Autodesk Inventor part; units mm, degrees
(part 3 of 4)
  line L1036 (-8.35, 24.45) -> (-11.15, 24.45)
  line L1037 (-11.15, 43.95) -> (-8.35, 43.95)
  line L1038 (-9.5, 42.651) -> (-9.5, 43.15)
  line L1039 (-10, 43.15) -> (-10, 42.517)
  line L1040 (-10, 43.15) -> (-9.5, 42.45) construction
  line L1041 (-10, 42.45) -> (-9.5, 43.15) construction
  arc A311 (-9.5, 42.651) -> (-9.433, 42.401) centre (-9, 42.651) ccw
  arc A312 (-10, 42.517) -> (-9.933, 42.267) centre (-9.5, 42.517) ccw
  line L1042 (-8.35, 43.95) -> (-8.35, 43.15)
  line L1043 (-8.35, 43.15) -> (-9.5, 43.15)
  line L1044 (-9.5, 43.15) -> (-10, 43.15)
  line L1045 (-9.75, 48.75) -> (-9.75, 43.95)
  line L1046 (-10, 43.15) -> (-11.15, 43.15)
  line L1047 (-11.15, 43.15) -> (-11.15, 43.95)
  line L1048 (-9.933, 22.767) -> (-2.2258, 9.4177)
  line L1049 (-1.7258, 9.5516) -> (-9.433, 22.901)
  line L1050 (-9.5335, 23.075) -> (-9.9665, 22.825)
  line L1051 (-9.9665, 22.825) -> (-1.6923, 9.4936) construction
  line L1052 (-2.1253, 9.2436) -> (-9.5335, 23.075) construction
  line L1053 (-9.5, 23.65) -> (-10, 23.65)
  line L1054 (-9.5, 23.151) -> (-9.5, 23.65)
  line L1055 (-10, 23.65) -> (-10, 23.017)
  line L1056 (-10, 23.65) -> (-9.5, 22.95) construction
  line L1057 (-10, 22.95) -> (-9.5, 23.65) construction
  line L1058 (-10, 22.95) -> (-9.5, 22.95)
  arc A313 (-9.5, 23.151) -> (-9.433, 22.901) centre (-9, 23.151) ccw
  arc A314 (-10, 23.017) -> (-9.933, 22.767) centre (-9.5, 23.017) ccw
  line L1059 (-0.2828, -49.3267) -> (2.4885, -54.1267)
  line L1060 (-0.2081, -55.5191) -> (0.2919, -52.6564) construction
  line L1061 (-0.2081, -52.6564) -> (0.2919, -55.5191) construction
  line L1062 (0.2919, -52.7233) -> (0.2919, -55.5191)
  circle A315 centre (0.0419, -55.5191) radius 0.75
  line L1063 (-0.2081, -55.5191) -> (-0.2081, -52.8573)
  arc A316 (-1.9445, -52.117) -> (-2.0115, -51.867) centre (-2.4445, -52.117) ccw
  arc A317 (-1.4445, -51.983) -> (-1.5115, -51.733) centre (-1.9445, -51.983) ccw
  arc A318 (-0.2081, -52.8573) -> (-0.2751, -52.6073) centre (-0.7081, -52.8573) ccw
  arc A319 (0.2919, -52.7233) -> (0.2249, -52.4733) centre (-0.2081, -52.7233) ccw
  line L1064 (2.089, -54.4347) -> (-0.3833, -49.1526) construction
  arc A320 (-0.3498, -49.0767) -> (-0.2828, -49.3267) centre (0.1502, -49.0767) ccw
  arc A321 (-0.8498, -49.2107) -> (-0.7828, -49.4607) centre (-0.3498, -49.2107) ccw
  arc A322 (-2.1588, -49.2107) -> (-2.0918, -49.4607) centre (-1.6588, -49.2107) ccw
  arc A323 (-1.6588, -49.0767) -> (-1.5918, -49.3267) centre (-1.1588, -49.0767) ccw
  line L1065 (-0.1746, -52.7814) -> (-1.6923, -49.1526) construction
  line L1066 (2.5555, -60.0187) -> (2.0555, -60.0187)
  circle A324 centre (2.3055, -60.0191) radius 0.75
  line L1067 (0.2919, -55.5191) -> (-0.2081, -55.5191)
  line L1068 (-4.2704, -49.3778) -> (-3.7751, -50.2357)
  line L1069 (-4.1686, -50.5541) -> (-4.3798, -49.1883) construction
  arc A325 (-4.3374, -49.1278) -> (-4.2704, -49.3778) centre (-3.8374, -49.1278) ccw
  arc A326 (-3.7081, -50.4857) -> (-3.7751, -50.2357) centre (-4.2081, -50.4857) ccw
  arc A327 (-3.4678, -49.2107) -> (-3.4008, -49.4607) centre (-2.9678, -49.2107) ccw
  arc A328 (-2.9678, -49.0767) -> (-2.9008, -49.3267) centre (-2.4678, -49.0767) ccw
  arc A329 (-4.2081, -50.6197) -> (-4.2751, -50.3697) centre (-4.7081, -50.6197) ccw
  arc A330 (2.5555, -54.3767) -> (2.4885, -54.1267) centre (2.0555, -54.3767) ccw
  arc A331 (2.0555, -54.5107) -> (1.9885, -54.2607) centre (1.5555, -54.5107) ccw
  line L1070 (-3.7081, -55.5191) -> (-4.2081, -55.5191)
  circle A332 centre (-3.9581, -55.5191) radius 0.75
  line L1071 (-1.9445, -60.0191) -> (-1.4445, -60.0191)
  circle A333 centre (-1.6945, -60.0191) radius 0.75
  line L1072 (-5.9445, -60.0191) -> (-5.4445, -60.0191)
  circle A334 centre (-5.6945, -60.0191) radius 0.75
  line L1073 (-8.35, -53.55) -> (-11.15, -53.55)
  line L1074 (-9.4445, -54.35) -> (-8.35, -54.35)
  line L1075 (-8.35, -54.35) -> (-8.35, -53.55)
  line L1076 (-11.15, -54.35) -> (-9.9295, -54.35)
  line L1077 (-11.15, -53.55) -> (-11.15, -54.35)
  line L1078 (-19.7751, -52.6073) -> (-21.5918, -49.4607)
  line L1079 (-23.2081, -50.4857) -> (-23.2081, -55.5191)
  line L1080 (-23.7081, -55.5191) -> (-23.7081, -50.6197)
  line L1081 (-23.7081, -55.5191) -> (-23.2081, -50.4326) construction
  line L1082 (-23.7081, -50.4326) -> (-23.2081, -55.5191) construction
  line L1083 (-22.9008, -49.4607) -> (-21.5115, -51.867)
  line L1084 (-20.9445, -60.0191) -> (-20.9445, -51.983)
  line L1085 (-21.4445, -51.916) -> (-20.9445, -60.0191) construction
  line L1086 (-21.4445, -60.0191) -> (-20.9445, -51.916) construction
  line L1087 (-21.4445, -52.117) -> (-21.4445, -60.0191)
  line L1088 (-24.3128, -49.4383) -> (-23.2356, -50.3041) construction
  line L1089 (-23.7751, -50.3697) -> (-24.2704, -49.5118)
  line L1090 (-25.5188, -49.4607) -> (-25.5115, -49.4733)
  line L1091 (-24.9445, -60.0191) -> (-24.9445, -49.5893)
  line L1092 (-25.4445, -49.7233) -> (-25.4445, -60.0191)
  line L1093 (-24.9445, -49.5223) -> (-25.4445, -60.0191) construction
  line L1094 (-24.9445, -60.0191) -> (-25.4445, -49.5223) construction
  line L1095 (-17.4445, -60.0187) -> (-17.4445, -54.5107)
  line L1096 (-16.9445, -54.3767) -> (-16.9445, -60.0187)
  line L1097 (-17.4445, -54.3101) -> (-16.9445, -60.0187) construction
  line L1098 (-17.4445, -60.0187) -> (-16.9445, -54.3101) construction
  line L1099 (-29.4295, -60.0191) -> (-29.4295, -54.35)
  line L1100 (-28.9445, -60.0191) -> (-29.4295, -60.0191)
  circle A335 centre (-29.1945, -60.0191) radius 0.75
  line L1101 (-29.4295, -60.0191) -> (-28.9832, -54.35) construction
  line L1102 (-29.4295, -54.35) -> (-28.9445, -54.35)
  line L1103 (-28.9445, -54.35) -> (-28.9445, -60.0191)
  line L1104 (-29.4295, -54.2285) -> (-28.9445, -60.0191) construction
  arc A336 (-24.9445, -49.5893) -> (-25.0115, -49.3393) centre (-25.4445, -49.5893) ccw
  arc A337 (-24.3374, -49.2618) -> (-24.2704, -49.5118) centre (-23.8374, -49.2618) ccw
  arc A338 (-25.0858, -49.0767) -> (-25.0188, -49.3267) centre (-24.5858, -49.0767) ccw
  arc A339 (-25.4445, -49.7233) -> (-25.5115, -49.4733) centre (-25.9445, -49.7233) ccw
  arc A340 (-25.5858, -49.2107) -> (-25.5188, -49.4607) centre (-25.0858, -49.2107) ccw
  line L1105 (-22.9343, -49.4026) -> (-20.978, -51.791) construction
  line L1106 (-21.0115, -51.733) -> (-22.4008, -49.3267)
  line L1107 (-21.411, -52.041) -> (-22.5013, -49.1526) construction
  line L1108 (-17.5115, -54.2607) -> (-20.2828, -49.4607)
  line L1109 (-22.9678, -49.2107) -> (-22.9678, -8.0651)
  line L1110 (-22.9678, -49.2776) -> (-22.4678, -7.8641) construction
  line L1111 (-22.9678, -7.8641) -> (-22.4678, -49.2776) construction
  line L1112 (-22.4678, -7.9311) -> (-22.4678, -49.0767)
  line L1113 (-21.6588, 9.1677) -> (-21.6588, -49.2107)
  line L1114 (-21.1588, -49.0767) -> (-21.1588, 9.3016)
  line L1115 (-21.6588, -49.2776) -> (-21.1588, 9.3686) construction
  line L1116 (-20.3498, -49.2107) -> (-20.3498, 26.4004)
  line L1117 (-19.8498, 26.5344) -> (-19.8498, -49.0767)
  line L1118 (-21.6588, 9.3686) -> (-21.1588, -49.2776) construction
  line L1119 (-21.6253, -49.4026) -> (-19.2416, -52.5314) construction
  line L1120 (-20.3163, -49.4026) -> (-16.978, -54.1847) construction
  line L1121 (-21.0918, -49.3267) -> (-19.2751, -52.4733)
  line L1122 (-25.5858, -42.4055) -> (-25.5858, -49.2107)
  line L1123 (-25.0858, -49.0767) -> (-25.0858, -42.2693)
  line L1124 (-25.5858, -49.2776) -> (-25.0858, -42.2012) construction
  line L1125 (-25.5858, -42.2012) -> (-25.0858, -49.2776) construction
  line L1126 (-29.4309, -35.7355) -> (-25.6549, -42.1519)
  line L1127 (-25.5513, -42.328) -> (-29.0345, -35.4232) construction
  line L1128 (-25.1549, -42.0157) -> (-28.9309, -35.5993)
  arc A341 (-25.5858, -42.4055) -> (-25.6549, -42.1519) centre (-26.0858, -42.4055) ccw
  arc A342 (-25.0858, -42.2693) -> (-25.1549, -42.0157) centre (-25.5858, -42.2693) ccw
  line L1129 (-29.4655, -35.6768) -> (-25.1203, -42.0744) construction
  arc A343 (-29.5, -35.4819) -> (-29.4309, -35.7355) centre (-29, -35.4819) ccw
  arc A344 (-29, -35.3457) -> (-28.9309, -35.5993) centre (-28.5, -35.3457) ccw
  line L1130 (-29, -35.3457) -> (-29, -34.85)
  line L1131 (-29.5, -35.55) -> (-29, -34.85) construction
  line L1132 (-29.5, -34.85) -> (-29, -35.55) construction
  line L1133 (-29, -34.85) -> (-29.5, -34.85)
  line L1134 (-29.5, -34.85) -> (-29.5, -35.4819)
  line L1135 (-25.0115, -49.3393) -> (-25.0188, -49.3267)
  line L1136 (-24.3374, -25.1978) -> (-24.3374, -49.2618)
  line L1137 (-23.8374, -49.1278) -> (-23.8374, -25.0639)
  line L1138 (-24.3374, -25.002) -> (-23.8374, -49.3098) construction
  line L1139 (-24.3374, -49.3098) -> (-23.8374, -25.002) construction
  arc A345 (-23.8374, -25.0639) -> (-23.9043, -24.814) centre (-24.3374, -25.0639) ccw
  arc A346 (-24.3374, -25.1978) -> (-24.4043, -24.9479) centre (-24.8374, -25.1978) ccw
  line L1140 (-30.65, -34.85) -> (-29.5, -34.85)
  line L1141 (-29, -34.85) -> (-27.85, -34.85)
  line L1142 (-30.65, -34.05) -> (-30.65, -34.85)
  line L1143 (-27.85, -34.05) -> (-30.65, -34.05)
  line L1144 (-27.85, -34.85) -> (-27.85, -34.05)
  arc A347 (-29.5, -15.983) -> (-29.4331, -16.2329) centre (-29, -15.983) ccw
  line L1145 (-29.0335, -15.9251) -> (-29.4665, -16.1749)
  line L1146 (-29.4331, -16.2329) -> (-24.4043, -24.9479)
  line L1147 (-29.4665, -16.1749) -> (-23.8679, -24.8771) construction
  line L1148 (-24.301, -25.127) -> (-29.0335, -15.9251) construction
  line L1149 (-23.9043, -24.814) -> (-28.9331, -16.099)
  line L1150 (-29.5, -16.05) -> (-29, -16.05)
  arc A348 (-29, -15.8491) -> (-28.9331, -16.099) centre (-28.5, -15.8491) ccw
  line L1151 (-29.25, -15.35) -> (-29.25, -16.05)
  line L1152 (-29.5, -15.35) -> (-29, -16.05) construction
  line L1153 (-29.5, -16.05) -> (-29, -15.35) construction
  line L1154 (-29, -15.35) -> (-29.5, -15.35)
  line L1155 (-30.65, -15.35) -> (-29.5, -15.35)
  line L1156 (-27.85, -14.55) -> (-30.65, -14.55)
  line L1157 (-30.65, -14.55) -> (-30.65, -15.35)
  line L1158 (-29.5, -15.35) -> (-29.5, -15.983)
  arc A349 (-22.4678, -7.9311) -> (-22.5348, -7.6811) centre (-22.9678, -7.9311) ccw
  arc A350 (-22.9678, -8.0651) -> (-23.0348, -7.8151) centre (-23.4678, -8.0651) ccw
  line L1159 (-29, -15.8491) -> (-29, -15.35)
  line L1160 (-29, -15.35) -> (-27.85, -15.35)
  line L1161 (-27.85, -15.35) -> (-27.85, -14.55)
  line L1162 (-29.433, 3.267) -> (-23.0348, -7.8151)
  line L1163 (-22.5348, -7.6811) -> (-28.933, 3.401)
  line L1164 (-29.0335, 3.575) -> (-29.4665, 3.325)
  line L1165 (-29.4665, 3.325) -> (-22.5013, -7.7391) construction
  line L1166 (-22.9343, -7.9891) -> (-29.0335, 3.575) construction
  line L1167 (-29.5, 3.45) -> (-29, 3.45)
  arc A351 (-29.5, 3.517) -> (-29.433, 3.267) centre (-29, 3.517) ccw
  line L1168 (-27.85, 4.15) -> (-27.85, 4.95)
  line L1169 (-29, 4.15) -> (-27.85, 4.15)
  line L1170 (-29, 3.651) -> (-29, 4.15)
  line L1171 (-29, 4.15) -> (-29.5, 4.15)
  arc A352 (-29, 3.651) -> (-28.933, 3.401) centre (-28.5, 3.651) ccw
  line L1172 (-29.5, 4.15) -> (-29.5, 3.517)
  line L1173 (-27.85, 4.95) -> (-30.65, 4.95)
  line L1174 (-30.65, 4.95) -> (-30.65, 4.15)
  line L1175 (-30.65, 4.15) -> (-29.5, 4.15)
  line L1176 (-21.6253, 9.2436) -> (-21.1923, 9.4936)
  arc A353 (-21.6588, 9.1677) -> (-21.7258, 9.4177) centre (-22.1588, 9.1677) ccw
  arc A354 (-21.1588, 9.3016) -> (-21.2258, 9.5516) centre (-21.6588, 9.3016) ccw
  line L1177 (-29.433, 42.267) -> (-20.4168, 26.6504)
  line L1178 (-20.3163, 26.4764) -> (-19.8833, 26.7264)
  line L1179 (-19.9168, 26.7844) -> (-28.933, 42.401)
  line L1180 (-29.4665, 42.325) -> (-19.8833, 26.7264) construction
  line L1181 (-20.3163, 26.4764) -> (-29.0335, 42.575) construction
  arc A355 (-19.8498, 26.5344) -> (-19.9168, 26.7844) centre (-20.3498, 26.5344) ccw
  arc A356 (-20.3498, 26.4004) -> (-20.4168, 26.6504) centre (-20.8498, 26.4004) ccw
  line L1182 (-29, 23.65) -> (-27.85, 23.65)
  line L1183 (-27.85, 23.65) -> (-27.85, 24.45)
  line L1184 (-30.65, 24.45) -> (-30.65, 23.65)
  line L1185 (-30.65, 23.65) -> (-29.5, 23.65)
  line L1186 (-27.85, 24.45) -> (-30.65, 24.45)
  line L1187 (-30.65, 43.95) -> (-27.85, 43.95)
  line L1188 (-29, 42.651) -> (-29, 43.15)
  line L1189 (-29.5, 43.15) -> (-29.5, 42.517)
  line L1190 (-29.5, 43.15) -> (-29, 42.45) construction
  line L1191 (-29.5, 42.45) -> (-29, 43.15) construction
  arc A357 (-29, 42.651) -> (-28.933, 42.401) centre (-28.5, 42.651) ccw
  arc A358 (-29.5, 42.517) -> (-29.433, 42.267) centre (-29, 42.517) ccw
  line L1192 (-27.85, 43.95) -> (-27.85, 43.15)
  line L1193 (-27.85, 43.15) -> (-29, 43.15)
  line L1194 (-29, 43.15) -> (-29.5, 43.15)
  line L1195 (-29.25, 48.75) -> (-29.25, 43.95)
  line L1196 (-29.5, 43.15) -> (-30.65, 43.15)
  line L1197 (-30.65, 43.15) -> (-30.65, 43.95)
  line L1198 (-29.433, 22.767) -> (-21.7258, 9.4177)
  line L1199 (-21.2258, 9.5516) -> (-28.933, 22.901)
  line L1200 (-29.0335, 23.075) -> (-29.4665, 22.825)
  line L1201 (-29.4665, 22.825) -> (-21.1923, 9.4936) construction
  line L1202 (-21.6253, 9.2436) -> (-29.0335, 23.075) construction
  line L1203 (-29, 23.65) -> (-29.5, 23.65)
  line L1204 (-29, 23.151) -> (-29, 23.65)
  line L1205 (-29.5, 23.65) -> (-29.5, 23.017)
  line L1206 (-29.5, 23.65) -> (-29, 22.95) construction
  line L1207 (-29.5, 22.95) -> (-29, 23.65) construction
  line L1208 (-29.5, 22.95) -> (-29, 22.95)
  arc A359 (-29, 23.151) -> (-28.933, 22.901) centre (-28.5, 23.151) ccw
  arc A360 (-29.5, 23.017) -> (-29.433, 22.767) centre (-29, 23.017) ccw
  line L1209 (-19.7828, -49.3267) -> (-17.0115, -54.1267)
  line L1210 (-19.7081, -55.5191) -> (-19.2081, -52.6564) construction
  line L1211 (-19.7081, -52.6564) -> (-19.2081, -55.5191) construction
  line L1212 (-19.2081, -52.7233) -> (-19.2081, -55.5191)
  circle A361 centre (-19.4581, -55.5191) radius 0.75
  line L1213 (-19.7081, -55.5191) -> (-19.7081, -52.8573)
  arc A362 (-21.4445, -52.117) -> (-21.5115, -51.867) centre (-21.9445, -52.117) ccw
  arc A363 (-20.9445, -51.983) -> (-21.0115, -51.733) centre (-21.4445, -51.983) ccw
  arc A364 (-19.7081, -52.8573) -> (-19.7751, -52.6073) centre (-20.2081, -52.8573) ccw
  arc A365 (-19.2081, -52.7233) -> (-19.2751, -52.4733) centre (-19.7081, -52.7233) ccw
  line L1214 (-17.411, -54.4347) -> (-19.8833, -49.1526) construction
  arc A366 (-19.8498, -49.0767) -> (-19.7828, -49.3267) centre (-19.3498, -49.0767) ccw
  arc A367 (-20.3498, -49.2107) -> (-20.2828, -49.4607) centre (-19.8498, -49.2107) ccw
  arc A368 (-21.6588, -49.2107) -> (-21.5918, -49.4607) centre (-21.1588, -49.2107) ccw
  arc A369 (-21.1588, -49.0767) -> (-21.0918, -49.3267) centre (-20.6588, -49.0767) ccw
  line L1215 (-19.6746, -52.7814) -> (-21.1923, -49.1526) construction
  line L1216 (-16.9445, -60.0187) -> (-17.4445, -60.0187)
  circle A370 centre (-17.1945, -60.0191) radius 0.75
  line L1217 (-19.2081, -55.5191) -> (-19.7081, -55.5191)
  line L1218 (-23.7704, -49.3778) -> (-23.2751, -50.2357)
  line L1219 (-23.6686, -50.5541) -> (-23.8798, -49.1883) construction
  arc A371 (-23.8374, -49.1278) -> (-23.7704, -49.3778) centre (-23.3374, -49.1278) ccw
  arc A372 (-23.2081, -50.4857) -> (-23.2751, -50.2357) centre (-23.7081, -50.4857) ccw
  arc A373 (-22.9678, -49.2107) -> (-22.9008, -49.4607) centre (-22.4678, -49.2107) ccw
  arc A374 (-22.4678, -49.0767) -> (-22.4008, -49.3267) centre (-21.9678, -49.0767) ccw
  arc A375 (-23.7081, -50.6197) -> (-23.7751, -50.3697) centre (-24.2081, -50.6197) ccw
  arc A376 (-16.9445, -54.3767) -> (-17.0115, -54.1267) centre (-17.4445, -54.3767) ccw
  arc A377 (-17.4445, -54.5107) -> (-17.5115, -54.2607) centre (-17.9445, -54.5107) ccw
  line L1220 (-23.2081, -55.5191) -> (-23.7081, -55.5191)
  circle A378 centre (-23.4581, -55.5191) radius 0.75
  line L1221 (-21.4445, -60.0191) -> (-20.9445, -60.0191)
  circle A379 centre (-21.1945, -60.0191) radius 0.75
  line L1222 (-25.4445, -60.0191) -> (-24.9445, -60.0191)
  circle A380 centre (-25.1945, -60.0191) radius 0.75
  line L1223 (-27.85, -53.55) -> (-30.65, -53.55)
  line L1224 (-28.9445, -54.35) -> (-27.85, -54.35)
  line L1225 (-27.85, -54.35) -> (-27.85, -53.55)
  line L1226 (-30.65, -54.35) -> (-29.4295, -54.35)
  line L1227 (-30.65, -53.55) -> (-30.65, -54.35)
  point P0 (27.85, 43.15)
  point P1 (38.4002, -11.3381)
  point P2 (39.8528, -51.7937)
  point P3 (41.3055, -57.1644)
  point P4 (39.0419, -54.0877)
  point P5 (38.0666, -50.967)
  point P6 (36.5438, -50.5968)
  point P7 (37.3055, -55.9676)
  point P8 (37.0912, -19.9545)
  point P9 (35.7822, -28.5709)
  point P10 (35.0419, -52.9758)
  point P11 (34.7258, -49.8712)
  point P12 (33.3055, -54.7707)
  point P13 (33.1642, -45.7394)
  point P14 (34.4126, -37.1559)
  point P15 (33.8251, 34.5257)
  point P16 (29.25, 42.8)
  point P17 (33.1706, 16.1593)
  point P18 (31.8328, -20.526)
  point P19 (31.2071, -38.8756)
  point P20 (32.5161, -2.2071)
  point P21 (29.25, 23.3)
  point P22 (29.25, -15.7)
  point P23 (29.25, -35.2)
  point P24 (29.3055, -57.0343)
  point P25 (29.1945, 57.0343)
  point P26 (21.1945, 55.9676)
  point P27 (17.1945, 57.1644)
  point P28 (25.1945, 54.7707)
  point P29 (23.4581, 52.9758)
  point P30 (23.7742, 49.8712)
  point P31 (18.6472, 51.7937)
  point P32 (19.4581, 54.0877)
  point P33 (21.9562, 50.5968)
  point P34 (20.4334, 50.967)
  point P35 (25.3358, 45.7394)
  point P36 (24.0874, 37.1559)
  point P37 (27.2929, 38.8756)
  point P38 (29.25, 35.2)
  point P39 (29.25, 15.7)
  point P40 (25.9839, 2.2071)
  point P41 (20.0998, 11.3381)
  point P42 (21.4088, 19.9545)
  point P43 (22.7178, 28.5709)
  point P44 (25.3294, -16.1593)
  point P45 (29.25, -23.3)
  point P46 (24.6749, -34.5257)
  point P47 (29.25, -42.8)
  point P48 (26.6672, 20.526)
  point P49 (9.6945, 57.0343)
  point P50 (1.6945, 55.9676)
  point P51 (-2.3055, 57.1644)
  point P52 (5.6945, 54.7707)
  point P53 (3.9581, 52.9758)
  point P54 (4.2742, 49.8712)
  point P55 (-0.8528, 51.7937)
  point P56 (-0.0419, 54.0877)
  point P57 (2.4562, 50.5968)
  point P58 (0.9334, 50.967)
  point P59 (5.8358, 45.7394)
  point P60 (4.5874, 37.1559)
  point P61 (7.7929, 38.8756)
  point P62 (9.75, 35.2)
  point P63 (9.75, 15.7)
  point P64 (6.4839, 2.2071)
  point P65 (0.5998, 11.3381)
  point P66 (1.9088, 19.9545)
  point P67 (3.2178, 28.5709)
  point P68 (5.8294, -16.1593)
  point P69 (9.75, -23.3)
  point P70 (5.1749, -34.5257)
  point P71 (9.75, -42.8)
  point P72 (7.1672, 20.526)
  point P73 (-9.8055, 57.0343)
  point P74 (-17.8055, 55.9676)
  point P75 (-21.8055, 57.1644)
  point P76 (-13.8055, 54.7707)
  point P77 (-15.5419, 52.9758)
  point P78 (-15.2258, 49.8712)
  point P79 (-20.3528, 51.7937)
  point P80 (-19.5419, 54.0877)
  point P81 (-17.0438, 50.5968)
  point P82 (-18.5666, 50.967)
  point P83 (-13.6642, 45.7394)
  point P84 (-14.9126, 37.1559)
  point P85 (-11.7071, 38.8756)
  point P86 (-9.75, 35.2)
  point P87 (-9.75, 15.7)
  point P88 (-13.0161, 2.2071)
  point P89 (-18.9002, 11.3381)
  point P90 (-17.5912, 19.9545)
  point P91 (-16.2822, 28.5709)
  point P92 (-13.6706, -16.1593)
  point P93 (-9.75, -23.3)
  point P94 (-14.3251, -34.5257)
  point P95 (-9.75, -42.8)
  point P96 (-12.3328, 20.526)
  point P97 (-29.3055, 57.0343)
  point P98 (-37.3055, 55.9676)
  point P99 (-41.3055, 57.1644)
  point P100 (-33.3055, 54.7707)
  point P101 (-35.0419, 52.9758)
  point P102 (-34.7258, 49.8712)
  point P103 (-39.8528, 51.7937)
  point P104 (-39.0419, 54.0877)
  point P105 (-36.5438, 50.5968)
  point P106 (-38.0666, 50.967)
  point P107 (-33.1642, 45.7394)
  point P108 (-34.4126, 37.1559)
  point P109 (-31.2071, 38.8756)
  point P110 (-29.25, 35.2)
  point P111 (-29.25, 15.7)
  point P112 (-32.5161, 2.2071)
  point P113 (-38.4002, 11.3381)
  point P114 (-37.0912, 19.9545)
  point P115 (-35.7822, 28.5709)
  point P116 (-33.1706, -16.1593)
  point P117 (-29.25, -23.3)
  point P118 (-33.8251, -34.5257)
  point P119 (-29.25, -42.8)
  point P120 (-31.8328, 20.526)
  point P121 (17.8055, -55.9676)
  point P122 (15.5419, -52.9758)
  point P123 (18.5666, -50.967)
  point P124 (17.0438, -50.5968)
  point P125 (13.8055, -54.7707)
  point P126 (9.8055, -57.0343)
  point P127 (17.5912, -19.9545)
  point P128 (18.9002, -11.3381)
  point P129 (13.6642, -45.7394)
  point P130 (11.7071, -38.8756)
  point P131 (9.75, -35.2)
  point P132 (16.2822, -28.5709)
  point P133 (14.9126, -37.1559)
  point P134 (12.3328, -20.526)
  point P135 (9.75, -15.7)
  point P136 (13.0161, -2.2071)
  point P137 (14.3251, 34.5257)
  point P138 (9.75, 42.8)
  point P139 (13.6706, 16.1593)
  point P140 (9.75, 23.3)
  point P141 (19.5419, -54.0877)
  point P142 (20.3528, -51.7937)
  point P143 (21.8055, -57.1644)
  point P144 (15.2258, -49.8712)
  point P145 (-1.6945, -55.9676)
  point P146 (-3.9581, -52.9758)
  point P147 (-0.9334, -50.967)
  point P148 (-2.4562, -50.5968)
  point P149 (-5.6945, -54.7707)
  point P150 (-9.6945, -57.0343)
  point P151 (-1.9088, -19.9545)
  point P152 (-0.5998, -11.3381)
  point P153 (-5.8358, -45.7394)
  point P154 (-7.7929, -38.8756)
  point P155 (-9.75, -35.2)
  point P156 (-3.2178, -28.5709)
  point P157 (-4.5874, -37.1559)
  point P158 (-7.1672, -20.526)
  point P159 (-9.75, -15.7)
  point P160 (-6.4839, -2.2071)
  point P161 (-5.1749, 34.5257)
  point P162 (-9.75, 42.8)
  point P163 (-5.8294, 16.1593)
  point P164 (-9.75, 23.3)
  point P165 (0.0419, -54.0877)
  point P166 (0.8528, -51.7937)
  point P167 (2.3055, -57.1644)
  point P168 (-4.2742, -49.8712)
  point P169 (-21.1945, -55.9676)
  point P170 (-23.4581, -52.9758)
  point P171 (-20.4334, -50.967)
  point P172 (-21.9562, -50.5968)
  point P173 (-25.1945, -54.7707)
  point P174 (-29.1945, -57.0343)
  point P175 (-21.4088, -19.9545)
  point P176 (-20.0998, -11.3381)
  point P177 (-25.3358, -45.7394)
  point P178 (-27.2929, -38.8756)
  point P179 (-29.25, -35.2)
  point P180 (-22.7178, -28.5709)
  point P181 (-24.0874, -37.1559)
  point P182 (-26.6672, -20.526)
  point P183 (-29.25, -15.7)
  point P184 (-25.9839, -2.2071)
  point P185 (-24.6749, 34.5257)
  point P186 (-29.25, 42.8)
  point P187 (-25.3294, 16.1593)
  point P188 (-29.25, 23.3)
  point P189 (-19.4581, -54.0877)
  point P190 (-18.6472, -51.7937)
  point P191 (-17.1945, -57.1644)
  point P192 (-23.7742, -49.8712)
  dimension "d149" = 0.5
  dimension "d150" = 0.5
  dimension "d151" = 0.5
  dimension "d152" = 0.5
  dimension "d153" = 0.5
  dimension "d154" = 0.5
  dimension "d155" = 0.5
  dimension "d157" = 0.5
  dimension "d161" = 1.5
  dimension "d162" = 1.5
  dimension "d163" = 1.5
  dimension "d164" = 1.5
  dimension "d165" = 1.5
  dimension "d166" = 1.5
  dimension "d180" = 0.5
  dimension "d184" = 0.5
  dimension "d185" = 0.5
  dimension "d186" = 0.5
  dimension "d188" = 0.5
  dimension "d189" = 0.5
  dimension "d190" = 0.5
  dimension "d191" = 0.5
  dimension "d192" = 0.5
  dimension "d193" = 0.5
  dimension "d194" = 0.5
  dimension "d195" = 0.5
  dimension "d196" = 0.5
  dimension "d197" = 0.5
  dimension "d198" = 0.5
  dimension "d199" = 0.5
  dimension "d201" = 0.5
  dimension "d433" = 0.5
  dimension "d434" = 0.5
  dimension "d435" = 0.5
  dimension "d436" = 0.5
  dimension "d437" = 0.5
  dimension "d438" = 0.5
  dimension "d439" = 0.5
  dimension "d440" = 0.5
  dimension "d441" = 1.5
  dimension "d442" = 1.5
  dimension "d443" = 1.5
  dimension "d444" = 1.5
  dimension "d445" = 1.5
  dimension "d446" = 1.5
  dimension "d447" = 0.5
  dimension "d448" = 0.5
  dimension "d449" = 0.5
  dimension "d450" = 0.5
  dimension "d451" = 0.5
  dimension "d452" = 0.5
  dimension "d453" = 0.5
  dimension "d454" = 0.5
  dimension "d455" = 0.5
  dimension "d456" = 0.5
  dimension "d457" = 0.5
  dimension "d458" = 0.5
  dimension "d459" = 0.5
  dimension "d460" = 0.5
  dimension "d461" = 0.5
  dimension "d462" = 0.5
  dimension "d463" = 0.5
  dimension "d464" = 0.5
  dimension "d465" = 0.5
  constraints: 2400 end point, 640 point on circle, 592 point on line, 368 centre point, 364 midpoint, 320 tangent, 190 parallel, 120 equal radius, 57 perpendicular, 20 horizontal, 6 coincident, 4 collinear, 4 vertical
  measures "d149" distance of L8.start L7.end
  measures "d150" distance of L13.start L12.end
  measures "d151" distance of L18.start L17.end
  measures "d152" distance of L22.start L21.end
  measures "d153" distance of L25.end L26.start
  measures "d154" distance of L28.end L27.end
  measures "d155" distance of L34.end L35.start
  measures "d157" distance of L44.start L43.end
  measures "d161" diameter of A6
  measures "d162" diameter of A7
  measures "d163" diameter of A8
  measures "d164" diameter of A9
  measures "d165" diameter of A10
  measures "d166" diameter of A11
  measures "d180" radius of A31
  measures "d184" distance of L66.end L66.start
  measures "d185" radius of A32
  measures "d186" distance of L78.end L79.start
  measures "d188" distance of L82.end L82.start
  measures "d189" radius of A36
  measures "d190" distance of L93.end L94.start
  measures "d191" distance of L97.end L98.start
  measures "d192" distance of L102.end L103.start
  measures "d193" radius of A38
  measures "d194" radius of A40
  measures "d195" radius of A42
  measures "d196" distance of L118.end L118.start
  measures "d197" distance of L123.end L123.start
  measures "d198" distance of L126.end L126.start
  measures "d199" distance of L132.end L133.start
  measures "d201" distance of L156.start L159.start
  measures "d433" distance of L820.start L914.end
  measures "d434" distance of L797.start L798.end
  measures "d435" distance of L911.start L910.end
  measures "d436" distance of L819.start L915.end
  measures "d437" distance of L805.end L807.start
  measures "d438" distance of L785.end L786.start
  measures "d439" distance of L818.end L815.start
  measures "d440" distance of L782.start L781.end
  measures "d441" diameter of A278
  measures "d442" diameter of A287
  measures "d443" diameter of A269
  measures "d444" diameter of A286
  measures "d445" diameter of A288
  measures "d446" diameter of A243
  measures "d447" radius of A284
  measures "d448" distance of L878.end L878.start
  measures "d449" radius of A263
  measures "d450" distance of L890.end L891.start
  measures "d451" distance of L901.end L902.start
  measures "d452" radius of A262
  measures "d453" distance of L847.end L848.start
  measures "d454" distance of L829.end L827.start
  measures "d455" distance of L865.end L866.start
  measures "d456" radius of A257
  measures "d457" radius of A253
  measures "d458" radius of A250
  measures "d459" distance of L906.end L907.start
  measures "d460" distance of L867.end L867.start
  measures "d461" distance of L850.end L850.start
  measures "d462" distance of L832.end L831.start
  measures "d463" distance of L803.start L804.start
  measures "d464" distance of L970.start L1064.end
  measures "d465" distance of L947.start L948.end
sketch "Sketch8" plane through (0, 0, 0) normal (0, 1, 0) x (1, 0, 0)
  circle A0 centre (29.25, 48.75) radius 2.8 construction
  circle A1 centre (29.25, 29.25) radius 2.8 construction
  circle A2 centre (29.25, 9.75) radius 2.8 construction
  circle A3 centre (29.25, -9.75) radius 2.8 construction
  circle A4 centre (29.25, -29.25) radius 2.8 construction
  circle A5 centre (29.25, -48.75) radius 2.8 construction
  circle A6 centre (9.75, 48.75) radius 2.8 construction
  circle A7 centre (-9.75, 48.75) radius 2.8 construction
  circle A8 centre (-29.25, 48.75) radius 2.8 construction
  line L0 (32.05, 48.75) -> (35.05, 48.75)
  line L1 (12.55, 48.75) -> (15.55, 48.75)
  line L2 (37.05, 49.5879) -> (37.05, 47.9121) construction
  line L3 (37.05, 47.9121) -> (35.05, 47.9121) construction
  line L4 (35.05, 47.9121) -> (35.05, 49.5879) construction
  line L5 (35.05, 49.5879) -> (37.05, 49.5879) construction
  line L6 (17.55, 49.5604) -> (17.55, 47.9396) construction
  line L7 (17.55, 47.9396) -> (15.55, 47.9396) construction
  line L8 (15.55, 47.9396) -> (15.55, 49.5604) construction
  line L9 (15.55, 49.5604) -> (17.55, 49.5604) construction
  line L10 (-1.8787, 49.5758) -> (-1.8787, 47.9242) construction
  line L11 (-1.8787, 47.9242) -> (-3.95, 47.9242) construction
  line L12 (-3.95, 47.9242) -> (-3.95, 49.5758) construction
  line L13 (-3.95, 49.5758) -> (-1.8787, 49.5758) construction
  line L14 (-21.45, 49.6827) -> (-21.45, 47.8173) construction
  line L15 (-21.45, 47.8173) -> (-23.45, 47.8173) construction
  line L16 (-23.45, 47.8173) -> (-23.45, 49.6827) construction
  line L17 (-23.45, 49.6827) -> (-21.45, 49.6827) construction
  line L18 (-6.95, 48.75) -> (-3.95, 48.75)
  line L19 (-26.45, 48.75) -> (-23.45, 48.75)
  line L20 (29.25, -48.75) -> (47.25, -48.75)
  line L21 (29.25, -29.25) -> (45.25, -29.25)
  line L22 (29.25, -9.75) -> (45.25, -9.75)
  line L23 (29.25, 9.75) -> (45.25, 9.75)
  line L24 (29.25, 48.75) -> (45.25, 48.75)
  line L25 (29.25, 29.25) -> (45.25, 29.25)
  line L26 (49.3294, -47.9996) -> (49.3294, -49.5004) construction
  line L27 (49.3294, -49.5004) -> (47.25, -49.5004) construction
  line L28 (47.25, -49.5004) -> (47.25, -47.9996) construction
  line L29 (47.25, -47.9996) -> (49.3294, -47.9996) construction
  line L30 (47.2921, -28.4996) -> (47.2921, -30.0004) construction
  line L31 (47.2921, -30.0004) -> (45.25, -30.0004) construction
  line L32 (45.25, -30.0004) -> (45.25, -28.4996) construction
  line L33 (45.25, -28.4996) -> (47.2921, -28.4996) construction
  line L34 (47.25, -8.9996) -> (47.25, -10.5004) construction
  line L35 (47.25, -10.5004) -> (45.25, -10.5004) construction
  line L36 (45.25, -10.5004) -> (45.25, -8.9996) construction
  line L37 (45.25, -8.9996) -> (47.25, -8.9996) construction
  line L38 (47.3343, 10.5004) -> (47.3343, 8.9996) construction
  line L39 (47.3343, 8.9996) -> (45.25, 8.9996) construction
  line L40 (45.25, 8.9996) -> (45.25, 10.5004) construction
  line L41 (45.25, 10.5004) -> (47.3343, 10.5004) construction
  line L42 (47.2921, 30.0004) -> (47.2921, 28.4996) construction
  line L43 (47.2921, 28.4996) -> (45.25, 28.4996) construction
  line L44 (45.25, 28.4996) -> (45.25, 30.0004) construction
  line L45 (45.25, 30.0004) -> (47.2921, 30.0004) construction
  line L46 (47.2565, 49.5004) -> (47.2565, 47.9996) construction
  line L47 (47.2565, 47.9996) -> (45.25, 47.9996) construction
  line L48 (45.25, 47.9996) -> (45.25, 49.5004) construction
  line L49 (45.25, 49.5004) -> (47.2565, 49.5004) construction
  line L50 (35.05, 49.6009) -> (37.05, 48.9267)
  line L51 (37.05, 48.9267) -> (37.05, 48.5993)
  line L52 (37.05, 48.5993) -> (35.05, 47.925)
  line L53 (35.05, 47.925) -> (35.05, 48.2054)
  line L54 (35.05, 48.2054) -> (35.6092, 48.387)
  line L55 (35.6092, 48.387) -> (35.6092, 49.1503)
  line L56 (35.6092, 49.1503) -> (35.05, 49.3318)
  line L57 (35.05, 49.3318) -> (35.05, 49.6009)
  line L58 (35.8361, 48.4599) -> (36.7777, 48.7694)
  line L59 (36.7777, 48.7694) -> (35.8361, 49.0774)
  line L60 (35.8361, 49.0774) -> (35.8361, 48.4599)
  line L61 (45.25, 48.2216) -> (45.25, 49.1973)
  line L62 (45.25, 49.1973) -> (45.4542, 49.1973)
  line L63 (45.4542, 49.1973) -> (45.4542, 48.8343)
  line L64 (45.4542, 48.8343) -> (46.7946, 48.8343)
  line L65 (46.7946, 48.8343) -> (46.7946, 49.1973)
  line L66 (46.7946, 49.1973) -> (46.9777, 49.1973)
  spline S0 degree 2 poles (46.9777, 49.1973) (46.9777, 48.9915) (47.0944, 48.797) (47.2565, 48.784) knots 0 0 0 1 2 2 2
  line L67 (47.2565, 48.784) -> (47.2565, 48.5766)
  line L68 (47.2565, 48.5766) -> (45.4542, 48.5766)
  line L69 (45.4542, 48.5766) -> (45.4542, 48.2216)
  line L70 (45.4542, 48.2216) -> (45.25, 48.2216)
  line L71 (45.25, 28.6212) -> (45.25, 29.8545)
  line L72 (45.25, 29.8545) -> (45.5336, 29.8545)
  spline S1 degree 2 poles (45.5336, 29.8545) (45.6584, 29.7216) (45.8902, 29.485) (46.015, 29.3716) knots 0 0 0 1 2 2 2
  spline S2 degree 2 poles (46.015, 29.3716) (46.2662, 29.143) (46.5677, 28.9761) (46.7281, 28.9761) knots 0 0 0 1 2 2 2
  spline S3 degree 2 poles (46.7281, 28.9761) (46.8124, 28.9761) (46.9388, 29.028) (46.9793, 29.075) knots 0 0 0 1 2 2 2
  spline S4 degree 2 poles (46.9793, 29.075) (47.0199, 29.122) (47.0604, 29.2451) (47.0604, 29.3197) knots 0 0 0 1 2 2 2
  spline S5 degree 2 poles (47.0604, 29.3197) (47.0604, 29.391) (47.0247, 29.5369) (46.9972, 29.6033) knots 0 0 0 1 2 2 2
  spline S6 degree 2 poles (46.9972, 29.6033) (46.9745, 29.66) (46.9096, 29.7654) (46.887, 29.7978) knots 0 0 0 1 2 2 2
  line L73 (46.887, 29.7978) -> (46.887, 29.8124)
  line L74 (46.887, 29.8124) -> (47.1722, 29.8124)
  spline S7 degree 2 poles (47.1722, 29.8124) (47.2127, 29.7297) (47.2921, 29.4331) (47.2921, 29.3002) knots 0 0 0 1 2 2 2
  spline S8 degree 2 poles (47.2921, 29.3002) (47.2921, 29.0199) (46.9955, 28.7038) (46.7427, 28.7038) knots 0 0 0 1 2 2 2
  spline S9 degree 2 poles (46.7427, 28.7038) (46.6244, 28.7038) (46.4267, 28.7589) (46.3424, 28.8075) knots 0 0 0 1 2 2 2
  spline S10 degree 2 poles (46.3424, 28.8075) (46.2549, 28.8562) (46.0831, 28.9972) (46.0004, 29.075) knots 0 0 0 1 2 2 2
  spline S11 degree 2 poles (46.0004, 29.075) (45.8626, 29.2014) (45.5677, 29.5109) (45.4818, 29.6033) knots 0 0 0 1 2 2 2
  line L75 (45.4818, 29.6033) -> (45.4818, 28.6212)
  line L76 (45.4818, 28.6212) -> (45.25, 28.6212)
  spline S12 degree 2 poles (47.1025, 9.8148) (47.1025, 9.8878) (47.0669, 10.032) (47.0393, 10.1017) knots 0 0 0 1 2 2 2
  spline S13 degree 2 poles (47.0393, 10.1017) (47.0118, 10.1665) (46.9534, 10.2622) (46.9275, 10.2994) knots 0 0 0 1 2 2 2
  line L77 (46.9275, 10.2994) -> (46.9275, 10.3156)
  line L78 (46.9275, 10.3156) -> (47.2111, 10.3156)
  spline S14 degree 2 poles (47.2111, 10.3156) (47.2581, 10.2281) (47.3343, 9.9283) (47.3343, 9.7938) knots 0 0 0 1 2 2 2
  spline S15 degree 2 poles (47.3343, 9.7938) (47.3343, 9.6576) (47.2792, 9.455) (47.2208, 9.3724) knots 0 0 0 1 2 2 2
  spline S16 degree 2 poles (47.2208, 9.3724) (47.1576, 9.2848) (46.9745, 9.1941) (46.8513, 9.1941) knots 0 0 0 1 2 2 2
  spline S17 degree 2 poles (46.8513, 9.1941) (46.686, 9.1941) (46.4364, 9.4113) (46.404, 9.5636) knots 0 0 0 1 2 2 2
  line L79 (46.404, 9.5636) -> (46.3845, 9.5636)
  spline S18 degree 2 poles (46.3845, 9.5636) (46.3716, 9.5004) (46.3132, 9.3562) (46.2549, 9.2946) knots 0 0 0 1 2 2 2
  spline S19 degree 2 poles (46.2549, 9.2946) (46.1981, 9.233) (46.0166, 9.1552) (45.8853, 9.1552) knots 0 0 0 1 2 2 2
  spline S20 degree 2 poles (45.8853, 9.1552) (45.7508, 9.1552) (45.5223, 9.2476) (45.4348, 9.3318) knots 0 0 0 1 2 2 2
  spline S21 degree 2 poles (45.4348, 9.3318) (45.344, 9.4194) (45.25, 9.6673) (45.25, 9.8246) knots 0 0 0 1 2 2 2
  spline S22 degree 2 poles (45.25, 9.8246) (45.25, 9.9753) (45.3229, 10.2703) (45.3732, 10.3707) knots 0 0 0 1 2 2 2
  line L80 (45.3732, 10.3707) -> (45.6568, 10.3707)
  line L81 (45.6568, 10.3707) -> (45.6568, 10.3513)
  spline S23 degree 2 poles (45.6568, 10.3513) (45.5952, 10.267) (45.4818, 9.9818) (45.4818, 9.8408) knots 0 0 0 1 2 2 2
  spline S24 degree 2 poles (45.4818, 9.8408) (45.4818, 9.7581) (45.5336, 9.5928) (45.5936, 9.5377) knots 0 0 0 1 2 2 2
  spline S25 degree 2 poles (45.5936, 9.5377) (45.6536, 9.4842) (45.7962, 9.4275) (45.9048, 9.4275) knots 0 0 0 1 2 2 2
  spline S26 degree 2 poles (45.9048, 9.4275) (46.0134, 9.4275) (46.1544, 9.4907) (46.1949, 9.5474) knots 0 0 0 1 2 2 2
  spline S27 degree 2 poles (46.1949, 9.5474) (46.2354, 9.6041) (46.2662, 9.7581) (46.2662, 9.8489) knots 0 0 0 1 2 2 2
  line L82 (46.2662, 9.8489) -> (46.2662, 9.9623)
  line L83 (46.2662, 9.9623) -> (46.4882, 9.9623)
  line L84 (46.4882, 9.9623) -> (46.4882, 9.8732)
  spline S28 degree 2 poles (46.4882, 9.8732) (46.4882, 9.6933) (46.66, 9.4664) (46.8237, 9.4664) knots 0 0 0 1 2 2 2
  spline S29 degree 2 poles (46.8237, 9.4664) (46.8999, 9.4664) (47.0085, 9.5247) (47.0409, 9.5717) knots 0 0 0 1 2 2 2
  spline S30 degree 2 poles (47.0409, 9.5717) (47.075, 9.622) (47.1025, 9.7451) (47.1025, 9.8148) knots 0 0 0 1 2 2 2
  line L85 (45.9372, -10.4323) -> (45.9372, -10.1941)
  line L86 (45.9372, -10.1941) -> (45.25, -10.1941)
  line L87 (45.25, -10.1941) -> (45.25, -9.9364)
  line L88 (45.25, -9.9364) -> (45.9372, -9.9364)
  line L89 (45.9372, -9.9364) -> (45.9372, -9.0531)
  line L90 (45.9372, -9.0531) -> (46.2192, -9.0531)
  line L91 (46.2192, -9.0531) -> (47.25, -9.9477)
  line L92 (47.25, -9.9477) -> (47.25, -10.1941)
  line L93 (47.25, -10.1941) -> (46.1528, -10.1941)
  line L94 (46.1528, -10.1941) -> (46.1528, -10.4323)
  line L95 (46.1528, -10.4323) -> (45.9372, -10.4323)
  line L96 (46.1528, -9.9364) -> (46.934, -9.9364)
  line L97 (46.934, -9.9364) -> (46.1528, -9.2638)
  line L98 (46.1528, -9.2638) -> (46.1528, -9.9364)
  spline S31 degree 2 poles (47.9404, -49.4096) (47.7865, -49.4096) (47.5255, -49.3075) (47.438, -49.2216) knots 0 0 0 1 2 2 2
  spline S32 degree 2 poles (47.438, -49.2216) (47.3456, -49.1325) (47.25, -48.9088) (47.25, -48.7743) knots 0 0 0 1 2 2 2
  spline S33 degree 2 poles (47.25, -48.7743) (47.25, -48.6398) (47.3408, -48.4177) (47.4315, -48.3335) knots 0 0 0 1 2 2 2
  spline S34 degree 2 poles (47.4315, -48.3335) (47.5401, -48.2297) (47.9048, -48.113) (48.1706, -48.113) knots 0 0 0 1 2 2 2
  spline S35 degree 2 poles (48.1706, -48.113) (48.4315, -48.113) (48.8513, -48.22) (49.0069, -48.3318) knots 0 0 0 1 2 2 2
  spline S36 degree 2 poles (49.0069, -48.3318) (49.1592, -48.4404) (49.3294, -48.784) (49.3294, -49.0093) knots 0 0 0 1 2 2 2
  spline S37 degree 2 poles (49.3294, -49.0093) (49.3294, -49.0758) (49.3165, -49.1925) (49.3019, -49.2362) knots 0 0 0 1 2 2 2
  line L99 (49.3019, -49.2362) -> (49.0442, -49.2362)
  line L100 (49.0442, -49.2362) -> (49.0442, -49.2249)
  spline S38 degree 2 poles (49.0442, -49.2249) (49.0636, -49.1876) (49.0976, -49.0515) (49.0976, -48.9737) knots 0 0 0 1 2 2 2
  spline S39 degree 2 poles (49.0976, -48.9737) (49.0976, -48.7241) (48.7605, -48.4177) (48.4299, -48.3886) knots 0 0 0 1 2 2 2
  spline S40 degree 2 poles (48.4299, -48.3886) (48.4964, -48.4842) (48.5693, -48.6852) (48.5693, -48.8051) knots 0 0 0 1 2 2 2
  spline S41 degree 2 poles (48.5693, -48.8051) (48.5693, -48.9218) (48.5223, -49.0968) (48.451, -49.1925) knots 0 0 0 1 2 2 2
  spline S42 degree 2 poles (48.451, -49.1925) (48.3683, -49.3027) (48.1122, -49.4096) (47.9404, -49.4096) knots 0 0 0 1 2 2 2
  spline S43 degree 2 poles (47.9291, -49.1374) (48.0523, -49.1374) (48.2192, -49.0725) (48.2776, -49.0012) knots 0 0 0 1 2 2 2
  spline S44 degree 2 poles (48.2776, -49.0012) (48.3197, -48.9477) (48.3472, -48.8148) (48.3472, -48.7451) knots 0 0 0 1 2 2 2
  spline S45 degree 2 poles (48.3472, -48.7451) (48.3472, -48.6511) (48.2905, -48.4745) (48.237, -48.3886) knots 0 0 0 1 2 2 2
  spline S46 degree 2 poles (48.237, -48.3886) (48.2079, -48.387) (48.1528, -48.3837) (48.1106, -48.3837) knots 0 0 0 1 2 2 2
  spline S47 degree 2 poles (48.1106, -48.3837) (47.9032, -48.3837) (47.6487, -48.4647) (47.5823, -48.5263) knots 0 0 0 1 2 2 2
  spline S48 degree 2 poles (47.5823, -48.5263) (47.519, -48.5831) (47.4688, -48.7062) (47.4688, -48.7759) knots 0 0 0 1 2 2 2
  spline S49 degree 2 poles (47.4688, -48.7759) (47.4688, -48.938) (47.6989, -49.1374) (47.9291, -49.1374) knots 0 0 0 1 2 2 2
  spline S50 degree 2 poles (45.9275, -29.8578) (45.7832, -29.8578) (45.5369, -29.7654) (45.4461, -29.6811) knots 0 0 0 1 2 2 2
  spline S51 degree 2 poles (45.4461, -29.6811) (45.3553, -29.5968) (45.25, -29.3456) (45.25, -29.19) knots 0 0 0 1 2 2 2
  spline S52 degree 2 poles (45.25, -29.19) (45.25, -29.0474) (45.3132, -28.7686) (45.3635, -28.6665) knots 0 0 0 1 2 2 2
  line L101 (45.3635, -28.6665) -> (45.6471, -28.6665)
  line L102 (45.6471, -28.6665) -> (45.6471, -28.686)
  spline S53 degree 2 poles (45.6471, -28.686) (45.6244, -28.7168) (45.566, -28.8318) (45.5401, -28.9015) knots 0 0 0 1 2 2 2
  spline S54 degree 2 poles (45.5401, -28.9015) (45.5126, -28.981) (45.4818, -29.1122) (45.4818, -29.1949) knots 0 0 0 1 2 2 2
  spline S55 degree 2 poles (45.4818, -29.1949) (45.4818, -29.2759) (45.5401, -29.4283) (45.6033, -29.4834) knots 0 0 0 1 2 2 2
  spline S56 degree 2 poles (45.6033, -29.4834) (45.6633, -29.5336) (45.8221, -29.5855) (45.9291, -29.5855) knots 0 0 0 1 2 2 2
  spline S57 degree 2 poles (45.9291, -29.5855) (46.0361, -29.5855) (46.1722, -29.5271) (46.2176, -29.472) knots 0 0 0 1 2 2 2
  spline S58 degree 2 poles (46.2176, -29.472) (46.2678, -29.4153) (46.31, -29.2468) (46.31, -29.1447) knots 0 0 0 1 2 2 2
  spline S59 degree 2 poles (46.31, -29.1447) (46.31, -29.0344) (46.2759, -28.8156) (46.2613, -28.7492) knots 0 0 0 1 2 2 2
  line L103 (46.2613, -28.7492) -> (47.2921, -28.7492)
  line L104 (47.2921, -28.7492) -> (47.2921, -29.8464)
  line L105 (47.2921, -29.8464) -> (47.0571, -29.8464)
  line L106 (47.0571, -29.8464) -> (47.0571, -29.0069)
  line L107 (47.0571, -29.0069) -> (46.5239, -29.0069)
  spline S60 degree 2 poles (46.5239, -29.0069) (46.5304, -29.0555) (46.5353, -29.1495) (46.5353, -29.1884) knots 0 0 0 1 2 2 2
  spline S61 degree 2 poles (46.5353, -29.1884) (46.5353, -29.3424) (46.485, -29.5547) (46.4105, -29.6519) knots 0 0 0 1 2 2 2
  spline S62 degree 2 poles (46.4105, -29.6519) (46.3359, -29.7508) (46.109, -29.8578) (45.9275, -29.8578) knots 0 0 0 1 2 2 2
  spline S63 degree 2 poles (16.1643, 48.0012) (16.0152, 48.0012) (15.7866, 48.1147) (15.7121, 48.2087) knots 0 0 0 1 2 2 2
  spline S64 degree 2 poles (15.7121, 48.2087) (15.6246, 48.3221) (15.55, 48.5798) (15.55, 48.784) knots 0 0 0 1 2 2 2
  line L108 (15.55, 48.784) -> (15.55, 49.3578)
  line L109 (15.55, 49.3578) -> (17.55, 49.3578)
  line L110 (17.55, 49.3578) -> (17.55, 48.8278)
  spline S65 degree 2 poles (17.55, 48.8278) (17.55, 48.6139) (17.5224, 48.3999) (17.469, 48.3027) knots 0 0 0 1 2 2 2
  spline S66 degree 2 poles (17.469, 48.3027) (17.4122, 48.1941) (17.2259, 48.0952) (17.0994, 48.0952) knots 0 0 0 1 2 2 2
  spline S67 degree 2 poles (17.0994, 48.0952) (16.9584, 48.0952) (16.7348, 48.2443) (16.6716, 48.3756) knots 0 0 0 1 2 2 2
  line L111 (16.6716, 48.3756) -> (16.6618, 48.3756)
  spline S68 degree 2 poles (16.6618, 48.3756) (16.6132, 48.1973) (16.3555, 48.0012) (16.1643, 48.0012) knots 0 0 0 1 2 2 2
  spline S69 degree 2 poles (16.1529, 48.2784) (16.2664, 48.2784) (16.4122, 48.3432) (16.4641, 48.4404) knots 0 0 0 1 2 2 2
  spline S70 degree 2 poles (16.4641, 48.4404) (16.4965, 48.5036) (16.516, 48.6528) (16.516, 48.7905) knots 0 0 0 1 2 2 2
  line L112 (16.516, 48.7905) -> (16.516, 49.092)
  line L113 (16.516, 49.092) -> (15.7769, 49.092)
  line L114 (15.7769, 49.092) -> (15.7769, 48.8764)
  spline S71 degree 2 poles (15.7769, 48.8764) (15.7769, 48.7014) (15.8093, 48.5004) (15.8612, 48.4226) knots 0 0 0 1 2 2 2
  spline S72 degree 2 poles (15.8612, 48.4226) (15.9147, 48.3481) (16.0476, 48.2784) (16.1529, 48.2784) knots 0 0 0 1 2 2 2
  spline S73 degree 2 poles (17.0622, 48.3724) (17.1335, 48.3724) (17.2404, 48.421) (17.2712, 48.4745) knots 0 0 0 1 2 2 2
  spline S74 degree 2 poles (17.2712, 48.4745) (17.3069, 48.5393) (17.3231, 48.6965) (17.3231, 48.8375) knots 0 0 0 1 2 2 2
  line L115 (17.3231, 48.8375) -> (17.3231, 49.092)
  line L116 (17.3231, 49.092) -> (16.738, 49.092)
  line L117 (16.738, 49.092) -> (16.738, 48.7905)
  spline S75 degree 2 poles (16.738, 48.7905) (16.738, 48.6657) (16.7639, 48.5474) (16.8045, 48.4842) knots 0 0 0 1 2 2 2
  spline S76 degree 2 poles (16.8045, 48.4842) (16.8434, 48.4226) (16.9682, 48.3724) (17.0622, 48.3724) knots 0 0 0 1 2 2 2
  spline S77 degree 2 poles (-3.95, 48.592) (-3.95, 48.7865) (-3.8187, 49.1155) (-3.6874, 49.2354) knots 0 0 0 1 2 2 2
  spline S78 degree 2 poles (-3.6874, 49.2354) (-3.5578, 49.3553) (-3.1688, 49.4866) (-2.916, 49.4866) knots 0 0 0 1 2 2 2
  spline S79 degree 2 poles (-2.916, 49.4866) (-2.6647, 49.4866) (-2.292, 49.3586) (-2.1542, 49.237) knots 0 0 0 1 2 2 2
  spline S80 degree 2 poles (-2.1542, 49.237) (-2.0197, 49.1171) (-1.8787, 48.7897) (-1.8787, 48.5871) knots 0 0 0 1 2 2 2
  spline S81 degree 2 poles (-1.8787, 48.5871) (-1.8787, 48.4866) (-1.9079, 48.31) (-1.9306, 48.2354) knots 0 0 0 1 2 2 2
  spline S82 degree 2 poles (-1.9306, 48.2354) (-1.9516, 48.1706) (-2.0116, 48.0361) (-2.0472, 47.9696) knots 0 0 0 1 2 2 2
  line L118 (-2.0472, 47.9696) -> (-2.3682, 47.9696)
  line L119 (-2.3682, 47.9696) -> (-2.3682, 47.9907)
  spline S83 degree 2 poles (-2.3682, 47.9907) (-2.3357, 48.0263) (-2.245, 48.1365) (-2.2012, 48.216) knots 0 0 0 1 2 2 2
  spline S84 degree 2 poles (-2.2012, 48.216) (-2.1591, 48.2921) (-2.1056, 48.472) (-2.1056, 48.5887) knots 0 0 0 1 2 2 2
  spline S85 degree 2 poles (-2.1056, 48.5887) (-2.1056, 48.7168) (-2.2109, 48.9453) (-2.3114, 49.0312) knots 0 0 0 1 2 2 2
  spline S86 degree 2 poles (-2.3114, 49.0312) (-2.4135, 49.1155) (-2.7231, 49.2095) (-2.916, 49.2095) knots 0 0 0 1 2 2 2
  spline S87 degree 2 poles (-2.916, 49.2095) (-3.1218, 49.2095) (-3.4184, 49.1106) (-3.5205, 49.0247) knots 0 0 0 1 2 2 2
  spline S88 degree 2 poles (-3.5205, 49.0247) (-3.6194, 48.9404) (-3.7199, 48.7152) (-3.7199, 48.5887) knots 0 0 0 1 2 2 2
  spline S89 degree 2 poles (-3.7199, 48.5887) (-3.7199, 48.4737) (-3.6631, 48.2776) (-3.621, 48.2014) knots 0 0 0 1 2 2 2
  spline S90 degree 2 poles (-3.621, 48.2014) (-3.5788, 48.1284) (-3.4913, 48.0199) (-3.4605, 47.9891) knots 0 0 0 1 2 2 2
  line L120 (-3.4605, 47.9891) -> (-3.4605, 47.9696)
  line L121 (-3.4605, 47.9696) -> (-3.7782, 47.9696)
  spline S91 degree 2 poles (-3.7782, 47.9696) (-3.809, 48.0361) (-3.8657, 48.1528) (-3.8917, 48.2354) knots 0 0 0 1 2 2 2
  spline S92 degree 2 poles (-3.8917, 48.2354) (-3.9208, 48.3229) (-3.95, 48.472) (-3.95, 48.592) knots 0 0 0 1 2 2 2
  spline S93 degree 2 poles (-22.4516, 47.9032) (-22.7255, 47.9032) (-23.1664, 48.1252) (-23.2895, 48.3116) knots 0 0 0 1 2 2 2
  spline S94 degree 2 poles (-23.2895, 48.3116) (-23.3852, 48.4639) (-23.45, 48.7767) (-23.45, 49.0199) knots 0 0 0 1 2 2 2
  line L122 (-23.45, 49.0199) -> (-23.45, 49.4801)
  line L123 (-23.45, 49.4801) -> (-21.45, 49.4801)
  line L124 (-21.45, 49.4801) -> (-21.45, 49.0247)
  spline S95 degree 2 poles (-21.45, 49.0247) (-21.45, 48.7427) (-21.5343, 48.4218) (-21.6088, 48.3083) knots 0 0 0 1 2 2 2
  spline S96 degree 2 poles (-21.6088, 48.3083) (-21.7369, 48.1155) (-22.1599, 47.9032) (-22.4516, 47.9032) knots 0 0 0 1 2 2 2
  spline S97 degree 2 poles (-22.4484, 48.1803) (-22.2182, 48.1803) (-21.8925, 48.3327) (-21.8001, 48.4834) knots 0 0 0 1 2 2 2
  spline S98 degree 2 poles (-21.8001, 48.4834) (-21.7369, 48.5904) (-21.6801, 48.8318) (-21.6801, 49.0118) knots 0 0 0 1 2 2 2
  line L125 (-21.6801, 49.0118) -> (-21.6801, 49.2143)
  line L126 (-21.6801, 49.2143) -> (-23.2199, 49.2143)
  line L127 (-23.2199, 49.2143) -> (-23.2199, 49.0118)
  spline S99 degree 2 poles (-23.2199, 49.0118) (-23.2199, 48.8351) (-23.1631, 48.5677) (-23.087, 48.4591) knots 0 0 0 1 2 2 2
  spline S100 degree 2 poles (-23.087, 48.4591) (-22.9929, 48.3197) (-22.6818, 48.1803) (-22.4484, 48.1803) knots 0 0 0 1 2 2 2
  point P0 (35.05, 48.75)
  point P1 (-23.45, 48.75)
  point P2 (15.55, 48.75)
  point P3 (45.25, 9.75)
  dimension "d355" = 3
  dimension "d356" = 3
  dimension "d358" = 3
  dimension "d359" = 3
  dimension "d360" = 18
  dimension "d361" = 16
  dimension "d362" = 16
  dimension "d363" = 16
  dimension "d364" = 16
  dimension "d365" = 16
  constraints: 20 end point, 10 horizontal, 10 midpoint, 1 coincident, 20 other
  measures "d355" distance of L0.start L0.end
  measures "d356" distance of L1.start L1.end
  measures "d358" distance of L18.start L18.end
  measures "d359" distance of L19.start L19.end
  measures "d360" distance of L20.start L20.end
  measures "d361" distance of L21.start L21.end
  measures "d362" distance of L22.start L22.end
  measures "d363" distance of L23.start L23.end
  measures "d364" distance of L24.start L24.end
  measures "d365" distance of L25.start L25.end
emboss "Emboss1" sketch "Sketch8" operation add depth 1 direction (0, -1, 0) contours L55 L56 L57 L50 L51 L24 L58 L59 L60 | L24 L60 L58 L51 L52 L53 L54 L55 | L61 L62 L63 L64 L65 L66 S0 L67 L68 L69 L70 | L71 L72 S1 S2 S3 S4 S5 S6 L73 L74 S7 S8 S9 S10 S11 L75 L76 | S12 S13 L77 L78 S14 S15 S16 S17 L79 S18 S19 S20 S21 S22 L80 L81 S23 S24 S25 S26 S27 L82 L83 L84 S28 S29 S30 | L85 L86 L87 L88 L89 L90 L91 L92 L93 L94 L95 | S31 S32 S33 S34 S35 S36 S37 L99 L100 S38 S39 S40 S41 S42 | S50 S51 S52 L101 L102 S53 S54 S55 S56 S57 S58 S59 L103 L104 L105 L106 L107 S60 S61 S62 | S63 S64 L108 L109 L110 S65 S66 S67 L111 S68 | S77 S78 S79 S80 S81 S82 L118 L119 S83 S84 S85 S86 S87 S88 S89 S90 L120 L121 S91 S92 | S93 S94 L122 L123 L124 S95 S96